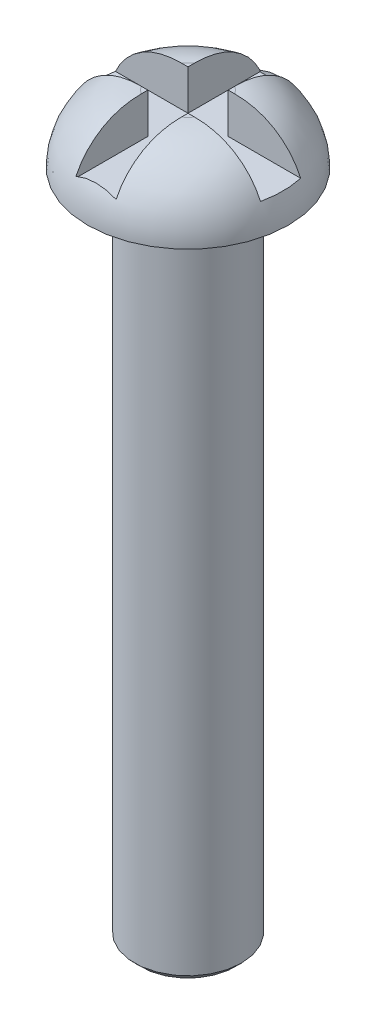
# Autodesk Inventor part: Vijs
Saved by Autodesk Inventor 2015 (Build 190159000, 159)
## iProperties
Created: 2016-04-19
Part Number: Vijs
Material: Generic
Document SubType Name: Modeling
Designer: david
Density: 1 g/cm^3
Appearance: Steel Galvanized
Author: david
Autodesk Inventor part; units mm, degrees
ref_plane "YZ Plane" through (0, 0, 0) normal (1, 0, 0) x (0, 1, 0)
ref_plane "XZ Plane" through (0, 0, 0) normal (0, 1, 0) x (-1, 0, 0)
ref_plane "XY Plane" through (0, 0, 0) normal (0, 0, 1) x (1, 0, 0)
sketch "Sketch1" plane through (0, 0, 0) normal (0, 1, 0) x (-1, 0, 0)
  circle A0 centre (0, 0) radius 4
  dimension "d0" = 8
  constraints: 1 centre point, 1 coincident
  measures "d0" diameter of A0
extrude "Extrusion1" add sketch "Sketch1" along normal blind 50
sketch "Sketch2" plane through (0, 50, 0) normal (0, 1, 0) x (1, 0, 0)
  circle A0 centre (0, 0) radius 7.5
  dimension "d3" = 15
  constraints: 1 centre point, 1 coincident
  measures "d3" diameter of A0
extrude "Extrusion2" add sketch "Sketch2" along normal blind 5
fillet "Fillet1" radius 5 1 edges at (-7.5, 55, 0)
sketch "Sketch3" plane through (0, 55, 0) normal (0, 1, 0) x (1, 0, 0)
  line L0 (7.4391, -1.5) -> (-7.4391, -1.5)
  line L1 (-7.4391, -1.5) -> (-7.4391, 1.5)
  line L2 (-7.4391, 1.5) -> (7.4391, 1.5)
  line L3 (7.4391, 1.5) -> (7.4391, -1.5)
  line L4 (7.4391, -1.5) -> (-7.4391, 1.5) construction
  line L5 (-7.4391, -1.5) -> (7.4391, 1.5) construction
  line L6 (1.5, -6.8733) -> (-1.5, -6.8733)
  line L7 (-1.5, -6.8733) -> (-1.5, 6.8733)
  line L8 (-1.5, 6.8733) -> (1.5, 6.8733)
  line L9 (1.5, 6.8733) -> (1.5, -6.8733)
  line L10 (1.5, -6.8733) -> (-1.5, 6.8733) construction
  line L11 (-1.5, -6.8733) -> (1.5, 6.8733) construction
  point P0 (0, 0)
  dimension "d7" = 3
  dimension "d8" = 3
  constraints: 24 end point, 4 midpoint, 4 parallel, 2 horizontal, 2 perpendicular
  measures "d7" distance of L0.end L1.end
  measures "d8" distance of L7.end L8.end
extrude "Extrusion3" cut sketch "Sketch3" against normal blind 3
thread "Thread1" size "M8x1.25" class "6g" standard "ANSI Metric M Profile" full length
chamfer "Chamfer1" distance 0.5 angle 45 1 edges at (4, 0, 0)
body "Solid1"
